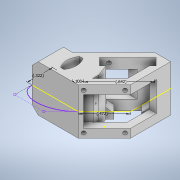
# Autodesk Inventor part: minimal micro scanner 3
Saved by Autodesk Inventor 2022 (Build 260153000, 153)
## iProperties
Created: 2023-08-23
Part Number: minimal micro scanner 3
Material: Generic
Document SubType Name: Modeling
Designer: William
Density: 1 g/cm^3
Appearance: Default
Author: William
Autodesk Inventor part; units mm, degrees
ref_plane "YZ Plane" through (0, 0, 0) normal (1, 0, 0) x (0, 1, 0)
ref_plane "XZ Plane" through (0, 0, 0) normal (0, 1, 0) x (-1, 0, 0)
ref_plane "XY Plane" through (0, 0, 0) normal (0, 0, 1) x (1, 0, 0)
sketch "Sketch1" plane through (0, 0, 0) normal (0, 1, 0) x (-1, 0, 0)
  line L0 (23.485281, -5.091169) -> (5.091169, -5.091169) construction
  line L1 (5.091169, -5.091169) -> (5.091169, -14.091169) construction
  line L2 (5.091169, -14.091169) -> (12.586501, -14.091169) construction
  line L3 (8.485281, 0) -> (0, -8.485281)
  line L4 (9.091169, -2.929646) -> (2.26066, -9.760155)
  line L5 (23.485281, 0) -> (23.485281, -8.191169)
  line L6 (0, -21.51579) -> (0, -8.485281)
  line L7 (5.091169, -5.091169) -> (4.242641, -4.242641) construction
  line L8 (1.2, -17.982338) -> (3.533452, -20.31579)
  line L9 (3.533452, -20.31579) -> (12.725841, -11.123402)
  line L10 (12.725841, -11.123402) -> (10.392388, -8.789949)
  line L11 (5.796194, -13.386144) -> (8.129646, -15.719596)
  line L12 (9.331728, -9.85061) -> (10.392388, -8.789949)
  line L13 (23.485281, -7.191169) -> (20.03151, -7.191169)
  line L14 (16.235281, -8.191169) -> (15.135281, -8.191169)
  line L15 (16.235281, -1.991169) -> (15.135281, -1.991169)
  arc A0 (15.135281, -1.991169) -> (15.135281, -8.191169) centre (19.440281, -5.091169) ccw
  arc A1 (16.235281, -8.191169) -> (16.235281, -1.991169) centre (11.930281, -5.091169) ccw
  line L16 (17.235281, -5.091169) -> (17.235281, -2.703822) construction
  line L17 (18.486501, -8.191169) -> (5.16188, -21.51579)
  line L18 (2.26066, -16.921677) -> (2.26066, -9.760155)
  line L19 (2.26066, -16.921677) -> (0, -16.921677)
  line L20 (9.369165, -2.65165) -> (7.601398, -0.883883)
  line L21 (3.55113, -15.631208) -> (5.884582, -17.96466)
  line L22 (5.884582, -17.96466) -> (10.37471, -13.474532)
  line L23 (10.37471, -13.474532) -> (8.041258, -11.14108)
  line L24 (9.091169, -2.929646) -> (9.369165, -2.65165)
  line L25 (8.485281, 0) -> (23.485281, 0)
  line L26 (5.16188, -21.51579) -> (0, -21.51579)
  line L27 (1.2, -17.982338) -> (3.55113, -15.631208)
  line L28 (8.041258, -11.14108) -> (9.331728, -9.85061)
  line L29 (18.03151, -5.291169) -> (17.23151, -5.291169)
  line L30 (23.485281, -5.091169) -> (17.235281, -5.091169)
  line L31 (7.929646, -4.091169) -> (7.929646, -6.091169)
  line L32 (7.929646, -5.091169) -> (14.135281, -5.091169)
  line L33 (7.929646, -5.291169) -> (8.729646, -5.291169)
  line L34 (7.929646, -6.091169) -> (9.331728, -9.85061)
  line L35 (8.041258, -11.14108) -> (3.55113, -15.631208) construction
  line L36 (14.48912, -3.186169) -> (16.881443, -3.186169)
  line L37 (14.48912, -6.996169) -> (16.881443, -6.996169)
  line L38 (15.685281, -3.186169) -> (15.685281, -6.996169) construction
  line L39 (8.729646, -5.291169) -> (14.48912, -6.996169)
  line L40 (20.03151, -7.191169) -> (18.03151, -5.291169)
  line L41 (23.485281, -8.191169) -> (18.486501, -8.191169)
  point P0 (0, 0)
  point P1 (6.929646, -5.091169)
  point P2 (15.685281, -8.191169)
  point P3 (21.185281, -5.091169)
  point P4 (14.139053, -5.291169)
  dimension "d0" = 45
  dimension "d2" = 2.5
  dimension "d5" = 6
  dimension "d6" = 6
  dimension "d11" = 9
  dimension "d12" = 3.3
  dimension "d13" = 13
  dimension "d46" = 1.5
  dimension "d56" = 2.1
  dimension "d58" = 5.09117
  dimension "d59" = 1.1
  dimension "d60" = 3.1
  dimension "d61" = 3.1
  dimension "d62" = 3.1
  dimension "d69" = 2.3
  dimension "d70" = 3.95
  dimension "d71" = 3.45377
  dimension "d73" = 1
  dimension "d93" = 1.2
  dimension "d97" = 1.5
  dimension "d101" = 4.75
  dimension "d102" = 1.2
  dimension "d103" = 135
  dimension "d104" = 45
  dimension "d109" = 2
  dimension "d112" = 1.2
  dimension "d113" = 0.8
  dimension "d114" = 0.2
  dimension "d115" = 2.8
  dimension "d116" = 15
  dimension "d117" = 3.81
  dimension "d118" = 6.35
  dimension "d123" = 2
  constraints: 84 end point, 14 perpendicular, 13 point on line, 12 point on circle, 8 horizontal, 7 midpoint, 6 parallel, 3 collinear, 3 equal length, 3 vertical, 2 centre point, 2 horizontal alignment, 2 vertical alignment, 1 equal radius, 1 tangent
  measures "d0" angle of L0 L4
  measures "d2" distance between parallel lines of L4 L3
  measures "d5" distance from line of L3.start L7
  measures "d6" distance from line of L3.end L7
  measures "d11" distance between parallel lines of L0 L2
  measures "d12" distance of L9.end L10.end
  measures "d13" distance of L8.end L9.end
  measures "d46" distance of L12.start L10.end
  measures "d56" distance between parallel lines of L0 L13
  measures "d58" distance of L5.start L0.start
  measures "d59" distance of L14.start L14.end
  measures "d60" distance between parallel lines of L0 L14
  measures "d61" distance between parallel lines of L0 L15
  measures "d69" distance from line of L5 point (21.185, -5.091)
  measures "d70" distance from line of point (21.185, -5.091) L16
  measures "d71" distance of L13.start L13.end
  measures "d73" distance of L5.end L13.start
  measures "d93" distance of L0.end L7.end
  measures "d97" distance of L8.start L18.start
  measures "d101" distance between parallel lines of L20 L7
  measures "d102" distance from line of L26 L8.end
  measures "d103" angle of L17 L26
  measures "d104" angle of L27 L19
  measures "d109" distance of L31.start L31.end
  measures "d112" distance from line of L6 L8.start
  measures "d113" distance of L33.start L33.end
  measures "d114" distance between parallel lines of L0 L33
  measures "d115" horizontal distance of L29.end L13.end
  measures "d116" distance of L3.start L5.start
  measures "d117" distance of L38.start L38.end
  measures "d118" distance of L23.end L21.start
  measures "d123" distance from line of L17 L9.end
sketch "Sketch5" plane through (0, 0, 0) normal (0, 1, 0) x (-1, 0, 0)
  line L0 (8.485281, 0) -> (0, -8.485281)
  line L1 (8.485281, 0) -> (23.485281, 0)
  line L2 (23.485281, 0) -> (23.485281, -8.191169)
  line L3 (23.485281, -8.191169) -> (18.486501, -8.191169)
  line L4 (18.486501, -8.191169) -> (5.16188, -21.51579)
  line L5 (5.16188, -21.51579) -> (0, -21.51579)
  line L6 (0, -21.51579) -> (0, -8.485281)
  line L7 (8.485281, 0) -> (14.072277, 5.586996) construction
  line L8 (14.072277, 5.586996) -> (23.485281, 5.586996) construction
  line L9 (23.485281, 5.586996) -> (23.485281, 0) construction
  spline S0 degree 3 poles (8.485281, 0) (14.072277, 5.586996) (23.485281, 5.586996) (23.485281, 0) knots 1 1 1 1 2 2 2 2
  line L10 (23.485281, -8.191169) -> (23.485281, -11.344104) construction
  line L11 (19.993376, -6.684293) -> (16.690449, -9.98722) construction
  spline S1 degree 4 poles (23.485281, -8.191169) (23.485281, -11.344104) (25.423174, -14.253772) (20.985891, -16.623756) (19.993376, -6.684293) (16.690449, -9.98722) knots 1 1 1 1 1 1.6974023 2 2 2 2 2
  line L12 (23.485281, -11.344104) -> (25.423174, -14.253772) construction
  line L13 (25.423174, -14.253772) -> (20.985891, -16.623756) construction
  line L14 (20.985891, -16.623756) -> (19.993376, -6.684293) construction
  point P0 (0, 0)
  dimension "d130" = 2.54
  dimension "d131" = 16.30386
  dimension "d132" = 8.19117
  dimension "d133" = 12
  constraints: 2 point on line, 1 collinear, 1 horizontal, 1 vertical, 6 other
  measures "d130" distance of L3.end L11.end
  measures "d131" distance of L4.end L11.end
  measures "d132" distance of L1.end L2.end
  measures "d133" distance of L0.start L0.end
extrude "Extrusion1" add sketch "Sketch1" along normal blind 7.5 and the other way blind 7.5 contours L25 L5 L30 A1 L15 A0 L32 L31 L4 L24 L20 L3 | L20 L24 L4 L18 L19 L6 L3 | L5 L13 L40 L29 A1 L30 | L19 L27 L8 L9 L10 L12 L34 L31 L33 L39 A0 L14 A1 L29 L40 L13 L5 L41 L17 L26 L6 | L27 L21 L9 L8 | L36 A0 L15 A1 | L32 A0 L39 L33 L31 | A1 L14 A0 L37 | L23 L28 L12 L10 L9
extrude "Extrusion11" cut sketch "Sketch1" along normal mid plane 9.5 contours L20 L24 L4 L18 L19 L6 L3
revolve "Revolution2" cut sketch "Sketch1" angle 360 about axis through (-23.485281, 0, -5.091169) along (1, 0, 0) contours L5 L13 L40 L29 A1 L30 | L32 A0 L39 L33 L31 | A1 L14 A0 L37
extrude "Extrusion3" cut sketch "Sketch1" along normal blind 13 contours A1 L37 A0 L36 | L27 L21 L9 L8 | L36 A0 L15 A1 | A1 L14 A0 L37 | L23 L28 L12 L10 L9
revolve "Revolution1" cut sketch "Sketch1" angle 360 about axis through (-5.796194, 0, -13.386144) along (-0.7071068, 0, -0.7071068) contours L27 L21 L9 L8
sketch "Sketch3" plane through (-1.737973, -5.5, -6.747309) normal (0.7071068, 0, 0.7071068) x (0.7071068, 0, -0.7071068)
  line L0 (-8.292136, -0.5) -> (1.207864, -0.5) construction
  line L1 (1.207864, -0.5) -> (1.207864, 11.5) construction
  line L2 (1.207864, 11.5) -> (-8.292136, 11.5) construction
  line L3 (-8.292136, 11.5) -> (-8.292136, -0.5) construction
  line L4 (-8.292136, 0.75) -> (1.207864, 0.75)
  line L5 (1.207864, 0.75) -> (1.207864, 10.25)
  line L6 (1.207864, 10.25) -> (-8.292136, 10.25)
  line L7 (-8.292136, 10.25) -> (-8.292136, 0.75)
  circle A0 centre (-8.292136, -0.5) radius 0.6
  circle A1 centre (-8.292136, 11.5) radius 0.6
  circle A2 centre (1.207864, -0.5) radius 0.6
  circle A3 centre (1.207864, 11.5) radius 0.6
  point P0 (-3.542136, 5.5)
  point P1 (-3.542136, 5.5)
  point P2 (-3.542136, 5.5)
  point P3 (-3.542136, 5.5)
  point P4 (1.207864, 5.5)
  point P5 (-3.542136, 11.5)
  point P6 (-3.542136, 0.75)
  point P7 (1.207864, 5.5)
  dimension "d37" = 12
  dimension "d38" = 1.2
  dimension "d95" = 9.5
  dimension "d96" = 9.5
  constraints: 16 end point, 4 centre point, 4 coincident, 4 midpoint, 4 parallel, 3 equal radius, 3 perpendicular, 2 horizontal, 2 horizontal alignment, 2 vertical alignment
  measures "d37" distance of L0.end L1.end
  measures "d38" diameter of A0
  measures "d95" distance of L1.end L2.end
  measures "d96" distance of L6.end L4.start
extrude "Extrusion6" cut sketch "Sketch3" against normal blind 2.7 contours L7 L6 L5 L4
extrude "Extrusion7" cut sketch "Sketch3" against normal blind 5 contours A0 | A1 | A2 | A3
sketch "Sketch4" plane through (-20.985891, -6.23, -5.691778) normal (-0.7071068, 0, -0.7071068) x (-0.7071068, 0, 0.7071068)
  line L0 (-7.378532, 1.98) -> (-16.378532, 1.98)
  line L1 (-16.378532, 1.98) -> (-16.378532, 10.48)
  line L2 (-16.378532, 10.48) -> (-7.378532, 10.48)
  line L3 (-7.378532, 10.48) -> (-7.378532, 1.98)
  circle A0 centre (-11.878532, 12.23) radius 0.6
  circle A1 centre (-11.878532, 0.23) radius 0.6
  line L4 (-17.178532, 6.23) -> (-11.878532, 6.23) construction
  line L5 (-22.378532, -1.27) -> (-22.378532, 13.73)
  point P0 (-16.378532, 6.23)
  point P1 (-11.878532, 10.48)
  point P2 (-11.878532, 1.98)
  point P3 (-7.378532, 6.23)
  dimension "d74" = 9
  dimension "d76" = 1.2
  dimension "d81" = 6
  dimension "d82" = 6
  dimension "d92" = 8.5
  dimension "d134" = 10.5
  constraints: 8 end point, 5 vertical alignment, 4 midpoint, 2 centre point, 2 parallel, 1 equal radius, 1 horizontal, 1 horizontal alignment, 1 perpendicular
  measures "d74" distance of L1.end L2.end
  measures "d76" diameter of A0
  measures "d81" distance of L4.end A0.centre
  measures "d82" distance of A1.centre L4.end
  measures "d92" distance of L2.end L0.start
  measures "d134" distance from line of L5 A0.centre
extrude "Extrusion8" cut sketch "Sketch4" against normal blind 4 contours A0 | A1
sketch "Sketch2" plane through (-23.485281, -7.5, 0) normal (-1, 0, 0) x (0, 0, 1)
  line L0 (-10.909188, 11.75) -> (-10.909188, 3.25)
  line L1 (-17.273149, 11.75) -> (-10.909188, 11.75)
  line L2 (-17.273149, 3.25) -> (-17.273149, 11.75)
  line L3 (-10.909188, 3.25) -> (-17.273149, 3.25)
  circle A0 centre (-5.091169, 7.5) radius 2.1
  circle A1 centre (-5.091169, 11.5) radius 0.6
  circle A2 centre (-5.091169, 3.5) radius 0.6
  circle A3 centre (-1.091169, 7.5) radius 0.6
  dimension "d83" = 4
  dimension "d84" = 1.2
  dimension "d85" = 4
  dimension "d86" = 4
  constraints: 3 centre point, 2 equal radius, 2 vertical alignment, 1 horizontal alignment
  measures "d83" distance of A0.centre A1.centre
  measures "d84" diameter of A1
  measures "d85" distance of A2.centre A0.centre
  measures "d86" distance of A3.centre A0.centre
extrude "Extrusion9" cut sketch "Sketch2" against normal up to next contours L0 L3 L2 L1
extrude "Extrusion10" cut sketch "Sketch2" against normal blind 3.5 contours A1 | A2 | A3
chamfer "Chamfer4" distance 2 angle 45 2 edges at (-23.4853, 7.5, -4.0956) (-23.4853, -7.5, -4.0956)
body "Solid1"
